Autodesk Inventor part; units mm, degrees
(part 2 of 2)
  measures "d114" diameter of A33
  measures "d115" diameter of A34
  measures "d116" diameter of A35
  measures "d117" diameter of A36
  measures "d118" diameter of A37
  measures "d119" diameter of A38
  measures "d120" diameter of A39
  measures "d121" diameter of A40
  measures "d122" diameter of A41
  measures "d123" diameter of A42
  measures "d124" diameter of A43
  measures "d125" diameter of A44
  measures "d126" diameter of A45
  measures "d127" diameter of A46
  measures "d128" diameter of A47
  measures "d129" diameter of A48
  measures "d130" diameter of A49
  measures "d131" diameter of A50
  measures "d132" diameter of A51
  measures "d133" diameter of A52
  measures "d134" diameter of A53
  measures "d135" diameter of A54
  measures "d136" diameter of A55
  measures "d137" diameter of A56
  measures "d138" diameter of A57
  measures "d139" diameter of A58
  measures "d140" diameter of A59
  measures "d141" diameter of A60
  measures "d142" diameter of A61
  measures "d143" diameter of A62
  measures "d144" diameter of A63
  measures "d145" diameter of A64
  measures "d146" diameter of A65
  measures "d147" diameter of A66
  measures "d148" diameter of A67
  measures "d149" diameter of A68
  measures "d150" diameter of A69
  measures "d151" diameter of A70
  measures "d152" diameter of A71
  measures "d155" diameter of A72
  measures "d156" diameter of A73
  measures "d264" diameter of A74
  measures "d265" diameter of A75
  measures "d267" distance between parallel lines of L17 L232
  measures "d268" diameter of A76
  measures "d269" diameter of A77
  measures "d270" diameter of A78
extrude "Extrusión2" add sketch "Boceto2" against normal up to surface (1.742 mm away)
sketch "Panel Shape" plane through (0, 0, 0) normal (0, 0, 1) x (1, 0, 0)
  line L0 (-22.8, -32.942) -> (-22.8, -37.5)
  arc A0 (-23.3, -38) -> (-22.8, -37.5) centre (-23.3, -37.5) ccw
  line L1 (-23.3, -38) -> (-29.8, -38)
  arc A1 (-30.3, -37.5) -> (-29.8, -38) centre (-29.8, -37.5) ccw
  line L2 (-30.3, -37.5) -> (-30.3, -31.2)
  arc A2 (-30.3, -31.2) -> (-30.8, -30.7) centre (-30.8, -31.2) ccw
  line L3 (-30.8, -30.7) -> (-76.8, -30.7)
  arc A3 (-76.8, -30.7) -> (-77.3, -31.2) centre (-76.8, -31.2) ccw
  line L4 (-77.3, -31.2) -> (-77.3, -49.2)
  arc A4 (-77.3, -49.2) -> (-75.3, -51.2) centre (-75.3, -49.2) ccw
  line L5 (-75.3, -51.2) -> (-71.048, -51.2)
  arc A5 (-65.048, -57.2) -> (-71.048, -51.2) centre (-71.048, -57.2) ccw
  line L6 (-65.048, -57.2) -> (-65.048, -62.7)
  arc A6 (-65.048, -62.7) -> (-63.048, -64.7) centre (-63.048, -62.7) ccw
  line L7 (-63.048, -64.7) -> (-30.8, -64.7)
  arc A7 (-30.8, -64.7) -> (-30.3, -64.2) centre (-30.8, -64.2) ccw
  line L8 (-30.3, -64.2) -> (-30.3, -59.8)
  arc A8 (-29.8, -59.3) -> (-30.3, -59.8) centre (-29.8, -59.8) ccw
  line L9 (-29.8, -59.3) -> (-23.3, -59.3)
  arc A9 (-22.8, -59.8) -> (-23.3, -59.3) centre (-23.3, -59.8) ccw
  line L10 (-22.8, -59.8) -> (-22.8, -62.458)
  arc A10 (-22.8, -62.458) -> (-22.3, -62.958) centre (-22.3, -62.458) ccw
  line L11 (-22.3, -62.958) -> (-16, -62.958)
  arc A11 (-16, -62.958) -> (-15.5, -62.458) centre (-16, -62.458) ccw
  line L12 (-15.5, -62.458) -> (-15.5, -60.4)
  arc A12 (25.5, -120.6) -> (26, -120.1) centre (25.5, -120.1) ccw
  line L13 (25.5, -120.6) -> (-25.5, -120.6)
  arc A13 (-26, -120.1) -> (-25.5, -120.6) centre (-25.5, -120.1) ccw
  line L14 (-26, -120.1) -> (-26, -66.6)
  arc A14 (-25.5, -66.1) -> (-26, -66.6) centre (-25.5, -66.6) ccw
  line L15 (-25.5, -66.1) -> (-16, -66.1)
  arc A15 (-15.5, -66.6) -> (-16, -66.1) centre (-16, -66.6) ccw
  line L16 (-15.5, -66.6) -> (-15.5, -72.9)
  arc A16 (-15.5, -72.9) -> (-15, -73.4) centre (-15, -72.9) ccw
  line L17 (-15, -59.9) -> (-13.5, -59.9)
  arc A17 (-13, -60.4) -> (-13.5, -59.9) centre (-13.5, -60.4) ccw
  line L18 (-13, -60.4) -> (-13, -72.9)
  arc A18 (-13.5, -73.4) -> (-13, -72.9) centre (-13.5, -72.9) ccw
  line L19 (-13.5, -73.4) -> (-15, -73.4)
  arc A19 (26, -73.9) -> (25.5, -73.4) centre (25.5, -73.9) ccw
  line L20 (26, -73.9) -> (26, -120.1)
  line L21 (7.4, 23.5) -> (7.4, 31.9)
  arc A20 (7.9, 32.4) -> (7.4, 31.9) centre (7.9, 31.9) ccw
  line L22 (7.9, 32.4) -> (12.55, 32.4)
  arc A21 (7.4, 23.5) -> (7.9, 23) centre (7.9, 23.5) ccw
  line L23 (7.9, 23) -> (25, 23)
  arc A22 (12.55, 32.4) -> (13.05, 32.9) centre (12.55, 32.9) ccw
  line L24 (13.05, 32.9) -> (13.05, 40.1)
  arc A23 (13.55, 40.6) -> (13.05, 40.1) centre (13.55, 40.1) ccw
  line L25 (13.55, 40.6) -> (36.8, 40.6)
  arc A24 (37.3, 40.1) -> (36.8, 40.6) centre (36.8, 40.1) ccw
  line L26 (37.3, 40.1) -> (37.3, 36)
  arc A25 (36.8, 35.5) -> (37.3, 36) centre (36.8, 36) ccw
  line L27 (36.8, 35.5) -> (34.4, 35.5)
  arc A26 (34.4, 35.5) -> (33.9, 35) centre (34.4, 35) ccw
  line L28 (33.9, 35) -> (33.9, 30.9)
  arc A27 (33.9, 30.9) -> (34.4, 30.4) centre (34.4, 30.9) ccw
  line L29 (38.9, 31.8) -> (38.9, 30.9)
  arc A28 (38.4, 30.4) -> (38.9, 30.9) centre (38.4, 30.9) ccw
  line L30 (38.4, 30.4) -> (34.4, 30.4)
  line L31 (77.3, 32.8) -> (77.3, 50.2)
  arc A29 (77.8, 50.7) -> (77.3, 50.2) centre (77.8, 50.2) ccw
  line L32 (77.8, 50.7) -> (79.8, 50.7)
  arc A30 (79.8, 50.7) -> (80.3, 51.2) centre (79.8, 51.2) ccw
  line L33 (80.3, 51.2) -> (80.3, 56.4)
  arc A31 (80.3, 56.4) -> (79.8, 56.9) centre (79.8, 56.4) ccw
  line L34 (79.8, 56.9) -> (58.9, 56.9)
  line L35 (54.4, 31.3) -> (57.9, 31.3)
  arc A32 (57.9, 31.3) -> (58.4, 31.8) centre (57.9, 31.8) ccw
  arc A33 (58.9, 32.3) -> (58.4, 31.8) centre (58.9, 31.8) ccw
  line L36 (58.9, 32.3) -> (76.8, 32.3)
  arc A34 (76.8, 32.3) -> (77.3, 32.8) centre (76.8, 32.8) ccw
  arc A35 (53.9, 31.8) -> (54.4, 31.3) centre (54.4, 31.8) ccw
  arc A36 (53.9, 31.8) -> (53.4, 32.3) centre (53.4, 31.8) ccw
  line L37 (53.4, 32.3) -> (39.4, 32.3)
  arc A37 (39.4, 32.3) -> (38.9, 31.8) centre (39.4, 31.8) ccw
  line L38 (36.8, 52) -> (13.55, 52)
  arc A38 (13.05, 52.5) -> (13.55, 52) centre (13.55, 52.5) ccw
  line L39 (13.05, 52.5) -> (13.05, 59.358)
  arc A39 (13.05, 59.358) -> (12.55, 59.858) centre (12.55, 59.358) ccw
  line L40 (12.55, 59.858) -> (-27.242, 59.858)
  arc A40 (36.8, 52) -> (37.3, 52.5) centre (36.8, 52.5) ccw
  line L41 (37.3, 52.5) -> (37.3, 53.2)
  arc A41 (-27.242, 59.858) -> (-27.742, 59.358) centre (-27.242, 59.358) ccw
  line L42 (-27.742, 59.358) -> (-27.742, 29.842)
  arc A42 (37.3, 53.2) -> (36.8, 53.7) centre (36.8, 53.2) ccw
  line L43 (36.8, 53.7) -> (34.4, 53.7)
  arc A43 (33.9, 54.2) -> (34.4, 53.7) centre (34.4, 54.2) ccw
  line L44 (33.9, 54.2) -> (33.9, 58.3)
  line L45 (-15, -26) -> (-13.5, -26)
  arc A44 (-13, -26.5) -> (-13.5, -26) centre (-13.5, -26.5) ccw
  line L46 (-13, -26.5) -> (-13, -35)
  arc A45 (-13.5, -35.5) -> (-13, -35) centre (-13.5, -35) ccw
  line L47 (-13.5, -35.5) -> (-15, -35.5)
  arc A46 (-15, -26) -> (-15.5, -26.5) centre (-15, -26.5) ccw
  line L48 (-15.5, -26.5) -> (-15.5, -28)
  arc A47 (-16, -28.5) -> (-15.5, -28) centre (-16, -28) ccw
  line L49 (-16, -28.5) -> (-25.5, -28.5)
  arc A48 (-26, -28) -> (-25.5, -28.5) centre (-25.5, -28) ccw
  line L50 (-26, -28) -> (-26, 25.5)
  arc A49 (-25.5, 26) -> (-26, 25.5) centre (-25.5, 25.5) ccw
  line L51 (-25.5, 26) -> (-20.6, 26)
  arc A50 (-20.1, 25.5) -> (-20.6, 26) centre (-20.6, 25.5) ccw
  line L52 (-20.1, 25.5) -> (-20.1, 23.5)
  arc A51 (-20.1, 23.5) -> (-19.6, 23) centre (-19.6, 23.5) ccw
  line L53 (-19.6, 32.4) -> (-18.3, 32.4)
  arc A52 (-17.8, 31.9) -> (-18.3, 32.4) centre (-18.3, 31.9) ccw
  line L54 (-17.8, 31.9) -> (-17.8, 23.5)
  arc A53 (-18.3, 23) -> (-17.8, 23.5) centre (-18.3, 23.5) ccw
  line L55 (-18.3, 23) -> (-19.6, 23)
  arc A54 (26, 22) -> (25, 23) centre (25, 22) ccw
  line L56 (26, 22) -> (26, -25.5)
  arc A55 (25.5, -26) -> (26, -25.5) centre (25.5, -25.5) ccw
  line L57 (-15.5, -35) -> (-15.5, -32.942)
  arc A56 (-15.5, -32.942) -> (-16, -32.442) centre (-16, -32.942) ccw
  line L58 (-16, -32.442) -> (-22.3, -32.442)
  arc A57 (-22.3, -32.442) -> (-22.8, -32.942) centre (-22.3, -32.942) ccw
  arc A58 (-15, -59.9) -> (-15.5, -60.4) centre (-15, -60.4) ccw
  arc A59 (25.5, -59.9) -> (26, -59.4) centre (25.5, -59.4) ccw
  line L59 (26, -59.4) -> (26, -36)
  arc A60 (26, -36) -> (25.5, -35.5) centre (25.5, -36) ccw
  arc A61 (-15.5, -35) -> (-15, -35.5) centre (-15, -35) ccw
  line L60 (25.5, -73.4) -> (25, -73.4)
  arc A62 (24.5, -72.9) -> (25, -73.4) centre (25, -72.9) ccw
  line L61 (24.5, -72.9) -> (24.5, -60.4)
  arc A63 (25, -59.9) -> (24.5, -60.4) centre (25, -60.4) ccw
  line L62 (25, -59.9) -> (25.5, -59.9)
  line L63 (24.5, -35) -> (24.5, -26.5)
  arc A64 (25, -26) -> (24.5, -26.5) centre (25, -26.5) ccw
  line L64 (25, -26) -> (25.5, -26)
  arc A65 (24.5, -35) -> (25, -35.5) centre (25, -35) ccw
  line L65 (25, -35.5) -> (25.5, -35.5)
  arc A66 (-27.742, 29.842) -> (-27.242, 29.342) centre (-27.242, 29.842) ccw
  line L66 (-27.242, 29.342) -> (-20.6, 29.342)
  arc A67 (-20.6, 29.342) -> (-20.1, 29.842) centre (-20.6, 29.842) ccw
  line L67 (-20.1, 29.842) -> (-20.1, 31.9)
  arc A68 (-19.6, 32.4) -> (-20.1, 31.9) centre (-19.6, 31.9) ccw
  arc A69 (34.4, 58.8) -> (33.9, 58.3) centre (34.4, 58.3) ccw
  arc A70 (58.4, 57.4) -> (58.9, 56.9) centre (58.9, 57.4) ccw
  arc A71 (58.4, 57.4) -> (57.9, 57.9) centre (57.9, 57.4) ccw
  line L68 (57.9, 57.9) -> (54.4, 57.9)
  arc A72 (54.4, 57.9) -> (53.9, 57.4) centre (54.4, 57.4) ccw
  arc A73 (53.4, 56.9) -> (53.9, 57.4) centre (53.4, 57.4) ccw
  line L69 (53.4, 56.9) -> (39.4, 56.9)
  arc A74 (38.9, 57.4) -> (39.4, 56.9) centre (39.4, 57.4) ccw
  line L70 (38.9, 57.4) -> (38.9, 58.3)
  arc A75 (38.9, 58.3) -> (38.4, 58.8) centre (38.4, 58.3) ccw
  line L71 (38.4, 58.8) -> (34.4, 58.8)
  circle A76 centre (-55.3, 51.4) radius 2.8
  circle A77 centre (58.3, 11.4) radius 2.8
  circle A78 centre (58.3, -43.6) radius 2.8
  circle A79 centre (58.3, -98.6) radius 2.8
  circle A80 centre (-55.3, -98.6) radius 2.8
  circle A81 centre (-55.3, -8.6) radius 2.8
  circle A82 centre (-20.3, -28.25) radius 0.25
  circle A83 centre (-19.3, -28.25) radius 0.25
  circle A84 centre (-18.3, -28.25) radius 0.25
  circle A85 centre (-19.3, -32.692) radius 0.25
  circle A86 centre (-18.3, -32.692) radius 0.25
  circle A87 centre (-20.3, -32.692) radius 0.25
  circle A88 centre (-28.25, -24.5) radius 0.25
  circle A89 centre (-25.75, -24.5) radius 0.25
  circle A90 centre (-25.75, -23.5) radius 0.25
  circle A91 centre (-25.75, -25.5) radius 0.25
  circle A92 centre (-28.25, -23.5) radius 0.25
  circle A93 centre (-28.25, -25.5) radius 0.25
  circle A94 centre (-28.25, -72.1) radius 0.25
  circle A95 centre (-25.75, -72.1) radius 0.25
  circle A96 centre (-25.75, -71.1) radius 0.25
  circle A97 centre (-25.75, -73.1) radius 0.25
  circle A98 centre (-28.25, -71.1) radius 0.25
  circle A99 centre (-28.25, -73.1) radius 0.25
  circle A100 centre (-36.3, -30.95) radius 0.25
  circle A101 centre (-36.3, -28.45) radius 0.25
  circle A102 centre (-37.3, -28.45) radius 0.25
  circle A103 centre (-35.3, -28.45) radius 0.25
  circle A104 centre (-37.3, -30.95) radius 0.25
  circle A105 centre (-35.3, -30.95) radius 0.25
  circle A106 centre (-71.3, -30.95) radius 0.25
  circle A107 centre (-71.3, -28.45) radius 0.25
  circle A108 centre (-72.3, -28.45) radius 0.25
  circle A109 centre (-70.3, -28.45) radius 0.25
  circle A110 centre (-72.3, -30.95) radius 0.25
  circle A111 centre (-70.3, -30.95) radius 0.25
  circle A112 centre (-59.05, -66.95) radius 0.25
  circle A113 centre (-59.05, -64.45) radius 0.25
  circle A114 centre (-60.05, -64.45) radius 0.25
  circle A115 centre (-58.05, -64.45) radius 0.25
  circle A116 centre (-60.05, -66.95) radius 0.25
  circle A117 centre (-58.05, -66.95) radius 0.25
  circle A118 centre (-36.3, -66.95) radius 0.25
  circle A119 centre (-36.3, -64.45) radius 0.25
  circle A120 centre (-37.3, -64.45) radius 0.25
  circle A121 centre (-35.3, -64.45) radius 0.25
  circle A122 centre (-37.3, -66.95) radius 0.25
  circle A123 centre (-35.3, -66.95) radius 0.25
  circle A124 centre (-19.3, -66.35) radius 0.25
  circle A125 centre (-19.3, -62.7) radius 0.25
  circle A126 centre (-20.3, -62.7) radius 0.25
  circle A127 centre (-18.3, -62.7) radius 0.25
  circle A128 centre (-20.3, -66.35) radius 0.25
  circle A129 centre (-18.3, -66.35) radius 0.25
  circle A130 centre (-25.75, -114.6) radius 0.25
  circle A131 centre (-28.25, -114.6) radius 0.25
  circle A132 centre (-28.25, -115.6) radius 0.25
  circle A133 centre (-28.25, -113.6) radius 0.25
  circle A134 centre (-25.75, -115.6) radius 0.25
  circle A135 centre (-25.75, -113.6) radius 0.25
  circle A136 centre (0, -120.35) radius 0.25
  circle A137 centre (0, -122.85) radius 0.25
  circle A138 centre (1, -122.85) radius 0.25
  circle A139 centre (-1, -122.85) radius 0.25
  circle A140 centre (1, -120.35) radius 0.25
  circle A141 centre (-1, -120.35) radius 0.25
  circle A142 centre (28.25, -114.6) radius 0.25
  circle A143 centre (25.75, -114.6) radius 0.25
  circle A144 centre (25.75, -115.6) radius 0.25
  circle A145 centre (25.75, -113.6) radius 0.25
  circle A146 centre (28.25, -115.6) radius 0.25
  circle A147 centre (28.25, -113.6) radius 0.25
  circle A148 centre (28.25, -82.8) radius 0.25
  circle A149 centre (25.75, -82.8) radius 0.25
  circle A150 centre (25.75, -83.8) radius 0.25
  circle A151 centre (25.75, -81.8) radius 0.25
  circle A152 centre (28.25, -83.8) radius 0.25
  circle A153 centre (28.25, -81.8) radius 0.25
  circle A154 centre (28.25, -20) radius 0.25
  circle A155 centre (25.75, -20) radius 0.25
  circle A156 centre (25.75, -21) radius 0.25
  circle A157 centre (25.75, -19) radius 0.25
  circle A158 centre (28.25, -21) radius 0.25
  circle A159 centre (28.25, -19) radius 0.25
  circle A160 centre (21, 22.75) radius 0.25
  circle A161 centre (21, 25.25) radius 0.25
  circle A162 centre (20, 25.25) radius 0.25
  circle A163 centre (22, 25.25) radius 0.25
  circle A164 centre (20, 22.75) radius 0.25
  circle A165 centre (22, 22.75) radius 0.25
  circle A166 centre (-25.75, 8.6) radius 0.25
  circle A167 centre (-28.25, 8.6) radius 0.25
  circle A168 centre (-28.25, 7.6) radius 0.25
  circle A169 centre (-28.25, 9.6) radius 0.25
  circle A170 centre (-25.75, 7.6) radius 0.25
  circle A171 centre (-25.75, 9.6) radius 0.25
  circle A172 centre (-27.492, 33.342) radius 0.25
  circle A173 centre (-27.492, 32.342) radius 0.25
  circle A174 centre (-27.492, 31.342) radius 0.25
  circle A175 centre (-29.992, 31.342) radius 0.25
  circle A176 centre (-29.992, 32.342) radius 0.25
  circle A177 centre (-29.992, 33.342) radius 0.25
  circle A178 centre (-29.992, 47.858) radius 0.25
  circle A179 centre (-27.492, 47.858) radius 0.25
  circle A180 centre (-29.992, 46.858) radius 0.25
  circle A181 centre (-29.992, 45.858) radius 0.25
  circle A182 centre (-27.492, 46.858) radius 0.25
  circle A183 centre (-27.492, 45.858) radius 0.25
  circle A184 centre (15.3, 36.6) radius 0.25
  circle A185 centre (15.3, 35.6) radius 0.25
  circle A186 centre (12.8, 34.6) radius 0.25
  circle A187 centre (12.8, 35.6) radius 0.25
  circle A188 centre (12.8, 36.6) radius 0.25
  circle A189 centre (15.3, 58) radius 0.25
  circle A190 centre (15.3, 57) radius 0.25
  circle A191 centre (15.3, 56) radius 0.25
  circle A192 centre (12.8, 56) radius 0.25
  circle A193 centre (12.8, 57) radius 0.25
  circle A194 centre (12.8, 58) radius 0.25
  circle A195 centre (28.25, -47.7) radius 0.25
  circle A196 centre (25.75, -47.7) radius 0.25
  circle A197 centre (25.75, -48.7) radius 0.25
  circle A198 centre (25.75, -46.7) radius 0.25
  circle A199 centre (28.25, -48.7) radius 0.25
  circle A200 centre (28.25, -46.7) radius 0.25
  circle A201 centre (25.75, -49.7) radius 0.25
  circle A202 centre (25.75, -45.7) radius 0.25
  circle A203 centre (28.25, -45.7) radius 0.25
  circle A204 centre (28.25, -49.7) radius 0.25
  circle A205 centre (47.7, 61.05) radius 0.25
  circle A206 centre (47.7, 56.65) radius 0.25
  circle A207 centre (48.7, 56.65) radius 0.25
  circle A208 centre (46.7, 56.65) radius 0.25
  circle A209 centre (48.7, 61.05) radius 0.25
  circle A210 centre (46.7, 61.05) radius 0.25
  circle A211 centre (69.7, 61.05) radius 0.25
  circle A212 centre (69.7, 56.65) radius 0.25
  circle A213 centre (70.7, 56.65) radius 0.25
  circle A214 centre (68.7, 56.65) radius 0.25
  circle A215 centre (70.7, 61.05) radius 0.25
  circle A216 centre (68.7, 61.05) radius 0.25
  circle A217 centre (69.7, 32.55) radius 0.25
  circle A218 centre (69.7, 28.15) radius 0.25
  circle A219 centre (70.7, 28.15) radius 0.25
  circle A220 centre (68.7, 28.15) radius 0.25
  circle A221 centre (70.7, 32.55) radius 0.25
  circle A222 centre (68.7, 32.55) radius 0.25
  circle A223 centre (47.7, 32.55) radius 0.25
  circle A224 centre (47.7, 28.15) radius 0.25
  circle A225 centre (48.7, 28.15) radius 0.25
  circle A226 centre (46.7, 28.15) radius 0.25
  circle A227 centre (48.7, 32.55) radius 0.25
  circle A228 centre (46.7, 32.55) radius 0.25
  circle A229 centre (-5.6, 62.108) radius 0.25
  circle A230 centre (-5.6, 59.608) radius 0.25
  circle A231 centre (-4.6, 59.608) radius 0.25
  circle A232 centre (-6.6, 59.608) radius 0.25
  circle A233 centre (-4.6, 62.108) radius 0.25
  circle A234 centre (-6.6, 62.108) radius 0.25
  circle A235 centre (23.035, -105.13) radius 0.37
  circle A236 centre (23.035, -106.4) radius 0.37
  circle A237 centre (23.035, -107.67) radius 0.37
  circle A238 centre (21.765, -105.13) radius 0.37
  circle A239 centre (21.765, -106.4) radius 0.37
  circle A240 centre (21.765, -107.67) radius 0.37
  circle A241 centre (23.035, -103.86) radius 0.37
  circle A242 centre (21.765, -103.86) radius 0.37
  circle A243 centre (23.035, -108.94) radius 0.37
  circle A244 centre (21.765, -108.94) radius 0.37
  circle A245 centre (-11.095, -17.035) radius 0.37
  circle A246 centre (-12.365, -17.035) radius 0.37
  circle A247 centre (-11.095, -15.765) radius 0.37
  circle A248 centre (-12.365, -15.765) radius 0.37
  circle A249 centre (-9.825, -17.035) radius 0.37
  circle A250 centre (-9.825, -15.765) radius 0.37
  circle A251 centre (-14.905, -17.035) radius 0.37
  circle A252 centre (-16.175, -17.035) radius 0.37
  circle A253 centre (-14.905, -15.765) radius 0.37
  circle A254 centre (-16.175, -15.765) radius 0.37
  circle A255 centre (-13.635, -17.035) radius 0.37
  circle A256 centre (-13.635, -15.765) radius 0.37
  circle A257 centre (21.465, -50.97) radius 0.37
  circle A258 centre (21.465, -49.7) radius 0.37
  circle A259 centre (21.465, -48.43) radius 0.37
  circle A260 centre (22.735, -50.97) radius 0.37
  circle A261 centre (22.735, -49.7) radius 0.37
  circle A262 centre (22.735, -48.43) radius 0.37
  circle A263 centre (21.465, -52.24) radius 0.37
  circle A264 centre (22.735, -52.24) radius 0.37
  circle A265 centre (21.465, -47.16) radius 0.37
  circle A266 centre (22.735, -47.16) radius 0.37
  circle A267 centre (73, 53.6) radius 1.5
  circle A268 centre (44.6, 35.6) radius 1.5
  circle A269 centre (44.6, 53.6) radius 1.5
  circle A270 centre (73, 35.6) radius 1.5
  circle A271 centre (15.3, 34.6) radius 0.25
  circle A272 centre (-36.6, -61.378) radius 2
  circle A273 centre (-36.6, -34.022) radius 2
  circle A274 centre (-19.1, -36.062) radius 2
  circle A275 centre (-23.092, 32.962) radius 2
  circle A276 centre (-9.192, 56.238) radius 2
  circle A277 centre (36.4, 56.256) radius 2
  circle A278 centre (78.021, 53.178) radius 2
  circle A279 centre (36.4, 32.98) radius 2
  circle A280 centre (56.15, 55.6) radius 2
  circle A281 centre (56.15, 33.6) radius 2
  circle A282 centre (-19.1, -59.338) radius 2
  circle A283 centre (-67.2, -34.022) radius 2
  circle A284 centre (-82.3, 64.858) radius 1.65
  circle A285 centre (85.3, 64.858) radius 1.65
  circle A286 centre (85.3, -125.6) radius 1.65
  circle A287 centre (-82.3, -125.6) radius 1.65
  arc A288 (31.4, 53.4) -> (31.9, 53.9) centre (31.4, 53.9) ccw
  line L72 (38.4, 58.8) -> (34.4, 58.8)
  line L73 (-76.8, -30.7) -> (-73.3, -30.7)
  line L74 (-79.3, -52.2) -> (-79.3, -29.7)
  arc A289 (-78.3, -28.7) -> (-79.3, -29.7) centre (-78.3, -29.7) ccw
  line L75 (-78.3, -28.7) -> (-73.3, -28.7)
  arc A290 (-73.3, -30.7) -> (-73.3, -28.7) centre (-73.3, -29.7) ccw
  arc A291 (-69.3, -28.7) -> (-69.3, -30.7) centre (-69.3, -29.7) ccw
  line L76 (-69.3, -28.7) -> (-38.3, -28.7)
  arc A292 (-38.3, -30.7) -> (-38.3, -28.7) centre (-38.3, -29.7) ccw
  arc A293 (-34.3, -28.7) -> (-34.3, -30.7) centre (-34.3, -29.7) ccw
  line L77 (-34.3, -28.7) -> (-28.5, -28.7)
  arc A294 (-28.5, -28.7) -> (-28, -28.2) centre (-28.5, -28.2) ccw
  line L78 (-28, -28.2) -> (-28, -26.3)
  arc A295 (-26, -26.3) -> (-28, -26.3) centre (-27, -26.3) ccw
  arc A296 (-28, -22.5) -> (-26, -22.5) centre (-27, -22.5) ccw
  line L79 (-28, -22.5) -> (-28, 6.6)
  arc A297 (-26, 6.6) -> (-28, 6.6) centre (-27, 6.6) ccw
  arc A298 (-28, 10.6) -> (-26, 10.6) centre (-27, 10.6) ccw
  line L80 (-28, 10.6) -> (-28, 26.842)
  arc A299 (-28, 26.842) -> (-28.5, 27.342) centre (-28.5, 26.842) ccw
  line L81 (-28.5, 27.342) -> (-28.742, 27.342)
  arc A300 (-29.742, 28.342) -> (-28.742, 27.342) centre (-28.742, 28.342) ccw
  line L82 (-29.742, 28.342) -> (-29.742, 30.342)
  arc A301 (-27.742, 30.342) -> (-29.742, 30.342) centre (-28.742, 30.342) ccw
  arc A302 (-29.742, 34.342) -> (-27.742, 34.342) centre (-28.742, 34.342) ccw
  line L83 (-29.742, 34.342) -> (-29.742, 44.858)
  arc A303 (-27.742, 44.858) -> (-29.742, 44.858) centre (-28.742, 44.858) ccw
  arc A304 (-29.742, 48.858) -> (-27.742, 48.858) centre (-28.742, 48.858) ccw
  line L84 (-29.742, 48.858) -> (-29.742, 60.858)
  arc A305 (-28.742, 61.858) -> (-29.742, 60.858) centre (-28.742, 60.858) ccw
  arc A306 (15.05, 60.858) -> (14.05, 61.858) centre (14.05, 60.858) ccw
  line L85 (15.05, 60.858) -> (15.05, 59)
  arc A307 (13.05, 59) -> (15.05, 59) centre (14.05, 59) ccw
  line L86 (31.4, 53.4) -> (15.55, 53.4)
  arc A308 (15.05, 53.9) -> (15.55, 53.4) centre (15.55, 53.9) ccw
  line L87 (15.05, 53.9) -> (15.05, 55)
  arc A309 (15.05, 55) -> (14.05, 56) centre (14.05, 55) ccw
  arc A310 (14.05, 56) -> (13.05, 55) centre (14.05, 55) ccw
  line L88 (13.05, 55) -> (13.05, 52.5)
  arc A311 (31.9, 29.4) -> (32.9, 28.4) centre (32.9, 29.4) ccw
  line L89 (31.9, 53.9) -> (31.9, 59.8)
  arc A312 (32.9, 60.8) -> (31.9, 59.8) centre (32.9, 59.8) ccw
  line L90 (32.9, 60.8) -> (45.7, 60.8)
  arc A313 (46.7, 59.8) -> (45.7, 60.8) centre (45.7, 59.8) ccw
  line L91 (46.7, 59.8) -> (46.7, 57.9)
  arc A314 (45.7, 56.9) -> (46.7, 57.9) centre (45.7, 57.9) ccw
  arc A315 (48.7, 57.9) -> (49.7, 56.9) centre (49.7, 57.9) ccw
  line L92 (48.7, 57.9) -> (48.7, 59.8)
  arc A316 (49.7, 60.8) -> (48.7, 59.8) centre (49.7, 59.8) ccw
  line L93 (49.7, 60.8) -> (67.7, 60.8)
  arc A317 (68.7, 59.8) -> (67.7, 60.8) centre (67.7, 59.8) ccw
  line L94 (68.7, 59.8) -> (68.7, 57.9)
  arc A318 (67.7, 56.9) -> (68.7, 57.9) centre (67.7, 57.9) ccw
  arc A319 (70.7, 57.9) -> (71.7, 56.9) centre (71.7, 57.9) ccw
  line L95 (70.7, 57.9) -> (70.7, 59.8)
  arc A320 (71.7, 60.8) -> (70.7, 59.8) centre (71.7, 59.8) ccw
  line L96 (71.7, 60.8) -> (81.3, 60.8)
  arc A321 (82.3, 59.8) -> (81.3, 60.8) centre (81.3, 59.8) ccw
  line L97 (82.3, 59.8) -> (82.3, 49.7)
  arc A322 (81.3, 48.7) -> (82.3, 49.7) centre (81.3, 49.7) ccw
  line L98 (81.3, 48.7) -> (80.3, 48.7)
  arc A323 (80.3, 48.7) -> (79.3, 47.7) centre (80.3, 47.7) ccw
  line L99 (79.3, 47.7) -> (79.3, 29.4)
  arc A324 (78.3, 28.4) -> (79.3, 29.4) centre (78.3, 29.4) ccw
  line L100 (78.3, 28.4) -> (71.7, 28.4)
  arc A325 (70.7, 29.4) -> (71.7, 28.4) centre (71.7, 29.4) ccw
  line L101 (70.7, 29.4) -> (70.7, 31.3)
  arc A326 (71.7, 32.3) -> (70.7, 31.3) centre (71.7, 31.3) ccw
  arc A327 (68.7, 31.3) -> (67.7, 32.3) centre (67.7, 31.3) ccw
  line L102 (68.7, 31.3) -> (68.7, 29.4)
  arc A328 (67.7, 28.4) -> (68.7, 29.4) centre (67.7, 29.4) ccw
  line L103 (67.7, 28.4) -> (49.7, 28.4)
  arc A329 (48.7, 29.4) -> (49.7, 28.4) centre (49.7, 29.4) ccw
  line L104 (48.7, 29.4) -> (48.7, 31.3)
  arc A330 (49.7, 32.3) -> (48.7, 31.3) centre (49.7, 31.3) ccw
  arc A331 (46.7, 31.3) -> (45.7, 32.3) centre (45.7, 31.3) ccw
  line L105 (46.7, 31.3) -> (46.7, 29.4)
  arc A332 (45.7, 28.4) -> (46.7, 29.4) centre (45.7, 29.4) ccw
  line L106 (45.7, 28.4) -> (32.9, 28.4)
  line L107 (-69.3, -30.7) -> (-38.3, -30.7)
  line L108 (31.9, 29.4) -> (31.9, 37.9)
  arc A333 (31.9, 37.9) -> (31.4, 38.4) centre (31.4, 37.9) ccw
  line L109 (31.4, 38.4) -> (15.55, 38.4)
  arc A334 (15.55, 38.4) -> (15.05, 37.9) centre (15.55, 37.9) ccw
  line L110 (15.05, 37.9) -> (15.05, 37.6)
  arc A335 (14.05, 36.6) -> (15.05, 37.6) centre (14.05, 37.6) ccw
  arc A336 (13.05, 37.6) -> (14.05, 36.6) centre (14.05, 37.6) ccw
  line L111 (13.05, 37.6) -> (13.05, 40.1)
  arc A337 (15.05, 33.6) -> (13.05, 33.6) centre (14.05, 33.6) ccw
  line L112 (15.05, 33.6) -> (15.058, 25.5)
  arc A338 (15.058, 25.5) -> (15.558, 25) centre (15.558, 25.5) ccw
  line L113 (15.558, 25) -> (19, 25)
  arc A339 (19, 23) -> (19, 25) centre (19, 24) ccw
  arc A340 (23, 25) -> (23, 23) centre (23, 24) ccw
  line L114 (23, 25) -> (27, 25)
  arc A341 (28, 24) -> (27, 25) centre (27, 24) ccw
  line L115 (28, 24) -> (28, -18)
  arc A342 (26, -18) -> (28, -18) centre (27, -18) ccw
  arc A343 (28, -22) -> (26, -22) centre (27, -22) ccw
  line L116 (28, -22) -> (28, -44.7)
  arc A344 (26, -44.7) -> (28, -44.7) centre (27, -44.7) ccw
  arc A345 (28, -50.7) -> (26, -50.7) centre (27, -50.7) ccw
  line L117 (28, -50.7) -> (28, -80.8)
  arc A346 (26, -80.8) -> (28, -80.8) centre (27, -80.8) ccw
  arc A347 (28, -84.8) -> (26, -84.8) centre (27, -84.8) ccw
  line L118 (28, -84.8) -> (28, -112.6)
  arc A348 (26, -112.6) -> (28, -112.6) centre (27, -112.6) ccw
  arc A349 (28, -116.6) -> (26, -116.6) centre (27, -116.6) ccw
  line L119 (28, -116.6) -> (28, -121.6)
  arc A350 (27, -122.6) -> (28, -121.6) centre (27, -121.6) ccw
  line L120 (27, -122.6) -> (2, -122.6)
  arc A351 (2, -120.6) -> (2, -122.6) centre (2, -121.6) ccw
  arc A352 (-2, -122.6) -> (-2, -120.6) centre (-2, -121.6) ccw
  line L121 (-2, -122.6) -> (-27, -122.6)
  arc A353 (-28, -121.6) -> (-27, -122.6) centre (-27, -121.6) ccw
  line L122 (-28, -121.6) -> (-28, -116.6)
  arc A354 (-26, -116.6) -> (-28, -116.6) centre (-27, -116.6) ccw
  arc A355 (-28, -112.6) -> (-26, -112.6) centre (-27, -112.6) ccw
  line L123 (-28, -112.6) -> (-28, -74.1)
  arc A356 (-26, -74.1) -> (-28, -74.1) centre (-27, -74.1) ccw
  arc A357 (-28, -70.1) -> (-26, -70.1) centre (-27, -70.1) ccw
  line L124 (-28, -70.1) -> (-28, -67.2)
  arc A358 (-28, -67.2) -> (-28.5, -66.7) centre (-28.5, -67.2) ccw
  line L125 (-28.5, -66.7) -> (-34.3, -66.7)
  arc A359 (-34.3, -64.7) -> (-34.3, -66.7) centre (-34.3, -65.7) ccw
  arc A360 (-38.3, -66.7) -> (-38.3, -64.7) centre (-38.3, -65.7) ccw
  line L126 (-38.3, -66.7) -> (-57.048, -66.7)
  arc A361 (-57.048, -64.7) -> (-57.048, -66.7) centre (-57.048, -65.7) ccw
  arc A362 (-61.048, -66.7) -> (-61.048, -64.7) centre (-61.048, -65.7) ccw
  line L127 (-61.048, -66.7) -> (-66.048, -66.7)
  arc A363 (-67.048, -65.7) -> (-66.048, -66.7) centre (-66.048, -65.7) ccw
  line L128 (-67.048, -65.7) -> (-67.048, -57.2)
  arc A364 (-67.048, -57.2) -> (-71.048, -53.2) centre (-71.048, -57.2) ccw
  line L129 (-71.048, -53.2) -> (-78.3, -53.2)
  arc A365 (-79.3, -52.2) -> (-78.3, -53.2) centre (-78.3, -52.2) ccw
  line L130 (-20.3, -29.5) -> (-20.3, -31.442)
  arc A366 (-21.3, -32.442) -> (-20.3, -31.442) centre (-21.3, -31.442) ccw
  arc A367 (-18.3, -31.442) -> (-17.3, -32.442) centre (-17.3, -31.442) ccw
  line L131 (-18.3, -31.442) -> (-18.3, -29.5)
  arc A368 (-17.3, -28.5) -> (-18.3, -29.5) centre (-17.3, -29.5) ccw
  arc A369 (-20.3, -29.5) -> (-21.3, -28.5) centre (-21.3, -29.5) ccw
  line L132 (-20.3, -63.958) -> (-20.3, -65.1)
  arc A370 (-21.3, -66.1) -> (-20.3, -65.1) centre (-21.3, -65.1) ccw
  arc A371 (-18.3, -65.1) -> (-17.3, -66.1) centre (-17.3, -65.1) ccw
  line L133 (-18.3, -65.1) -> (-18.3, -63.958)
  arc A372 (-17.3, -62.958) -> (-18.3, -63.958) centre (-17.3, -63.958) ccw
  arc A373 (-20.3, -63.958) -> (-21.3, -62.958) centre (-21.3, -63.958) ccw
  line L134 (-22.8, -32.942) -> (-22.8, -37.5)
  arc A374 (-23.3, -38) -> (-22.8, -37.5) centre (-23.3, -37.5) ccw
  line L135 (-23.3, -38) -> (-29.8, -38)
  arc A375 (-30.3, -37.5) -> (-29.8, -38) centre (-29.8, -37.5) ccw
  line L136 (-30.3, -37.5) -> (-30.3, -31.2)
  arc A376 (-30.3, -31.2) -> (-30.8, -30.7) centre (-30.8, -31.2) ccw
  arc A377 (-76.8, -30.7) -> (-77.3, -31.2) centre (-76.8, -31.2) ccw
  line L137 (-77.3, -31.2) -> (-77.3, -49.2)
  arc A378 (-77.3, -49.2) -> (-75.3, -51.2) centre (-75.3, -49.2) ccw
  line L138 (-75.3, -51.2) -> (-71.048, -51.2)
  arc A379 (-65.048, -57.2) -> (-71.048, -51.2) centre (-71.048, -57.2) ccw
  line L139 (-65.048, -57.2) -> (-65.048, -62.7)
  arc A380 (-65.048, -62.7) -> (-63.048, -64.7) centre (-63.048, -62.7) ccw
  arc A381 (-30.8, -64.7) -> (-30.3, -64.2) centre (-30.8, -64.2) ccw
  line L140 (-30.3, -64.2) -> (-30.3, -59.8)
  arc A382 (-29.8, -59.3) -> (-30.3, -59.8) centre (-29.8, -59.8) ccw
  line L141 (-29.8, -59.3) -> (-23.3, -59.3)
  arc A383 (-22.8, -59.8) -> (-23.3, -59.3) centre (-23.3, -59.8) ccw
  line L142 (-22.8, -59.8) -> (-22.8, -62.458)
  arc A384 (-22.8, -62.458) -> (-22.3, -62.958) centre (-22.3, -62.458) ccw
  arc A385 (-16, -62.958) -> (-15.5, -62.458) centre (-16, -62.458) ccw
  line L143 (-15.5, -62.458) -> (-15.5, -60.4)
  arc A386 (25.5, -120.6) -> (26, -120.1) centre (25.5, -120.1) ccw
  arc A387 (-26, -120.1) -> (-25.5, -120.6) centre (-25.5, -120.1) ccw
  arc A388 (-25.5, -66.1) -> (-26, -66.6) centre (-25.5, -66.6) ccw
  arc A389 (-15.5, -66.6) -> (-16, -66.1) centre (-16, -66.6) ccw
  line L144 (-15.5, -66.6) -> (-15.5, -72.9)
  arc A390 (-15.5, -72.9) -> (-15, -73.4) centre (-15, -72.9) ccw
  line L145 (-15, -59.9) -> (-13.5, -59.9)
  arc A391 (-13, -60.4) -> (-13.5, -59.9) centre (-13.5, -60.4) ccw
  line L146 (-13, -60.4) -> (-13, -72.9)
  arc A392 (-13.5, -73.4) -> (-13, -72.9) centre (-13.5, -72.9) ccw
  line L147 (-13.5, -73.4) -> (-15, -73.4)
  arc A393 (26, -73.9) -> (25.5, -73.4) centre (25.5, -73.9) ccw
  line L148 (7.4, 23.5) -> (7.4, 31.9)
  arc A394 (7.9, 32.4) -> (7.4, 31.9) centre (7.9, 31.9) ccw
  line L149 (7.9, 32.4) -> (12.55, 32.4)
  arc A395 (7.4, 23.5) -> (7.9, 23) centre (7.9, 23.5) ccw
  arc A396 (12.55, 32.4) -> (13.05, 32.9) centre (12.55, 32.9) ccw
  arc A397 (13.55, 40.6) -> (13.05, 40.1) centre (13.55, 40.1) ccw
  line L150 (13.55, 40.6) -> (36.8, 40.6)
  arc A398 (37.3, 40.1) -> (36.8, 40.6) centre (36.8, 40.1) ccw
  line L151 (37.3, 40.1) -> (37.3, 36)
  arc A399 (36.8, 35.5) -> (37.3, 36) centre (36.8, 36) ccw
  line L152 (36.8, 35.5) -> (34.4, 35.5)
  arc A400 (34.4, 35.5) -> (33.9, 35) centre (34.4, 35) ccw
  line L153 (33.9, 35) -> (33.9, 30.9)
  line L154 (-61.048, -64.7) -> (-63.048, -64.7)
  line L155 (-38.3, -64.7) -> (-57.048, -64.7)
  line L156 (-34.3, -64.7) -> (-30.8, -64.7)
  line L157 (-25.5, -66.1) -> (-21.3, -66.1)
  line L158 (-17.3, -66.1) -> (-16, -66.1)
  line L159 (-22.3, -62.958) -> (-21.3, -62.958)
  line L160 (-17.3, -62.958) -> (-16, -62.958)
  line L161 (-26, -112.6) -> (-26, -74.1)
  line L162 (-26, -120.1) -> (-26, -116.6)
  line L163 (-2, -120.6) -> (-25.5, -120.6)
  line L164 (25.5, -120.6) -> (2, -120.6)
  line L165 (26, -116.6) -> (26, -120.1)
  line L166 (26, -84.8) -> (26, -112.6)
  line L167 (26, -73.9) -> (26, -80.8)
  line L168 (26, -50.7) -> (26, -59.4)
  line L169 (-26, -70.1) -> (-26, -66.6)
  line L170 (-34.3, -30.7) -> (-30.8, -30.7)
  line L171 (-26, -28) -> (-26, -26.3)
  line L172 (-25.5, -28.5) -> (-21.3, -28.5)
  line L173 (-22.3, -32.442) -> (-21.3, -32.442)
  line L174 (-17.3, -32.442) -> (-16, -32.442)
  line L175 (-17.3, -28.5) -> (-16, -28.5)
  line L176 (26, -36) -> (26, -44.7)
  line L177 (26, -22) -> (26, -25.5)
  line L178 (26, 22) -> (26, -18)
  line L179 (23, 23) -> (25, 23)
  line L180 (7.9, 23) -> (19, 23)
  line L181 (13.05, 32.9) -> (13.05, 33.6)
  line L182 (-26, -22.5) -> (-26, 6.6)
  line L183 (-26, 10.6) -> (-26, 25.5)
  line L184 (-27.742, 29.842) -> (-27.742, 30.342)
  line L185 (-27.742, 34.342) -> (-27.742, 44.858)
  line L186 (-27.742, 48.858) -> (-27.742, 59.358)
  line L187 (13.05, 59.358) -> (13.05, 59)
  line L188 (39.4, 56.9) -> (45.7, 56.9)
  line L189 (49.7, 56.9) -> (53.4, 56.9)
  line L190 (58.9, 56.9) -> (67.7, 56.9)
  line L191 (71.7, 56.9) -> (79.8, 56.9)
  line L192 (45.7, 32.3) -> (39.4, 32.3)
  line L193 (53.4, 32.3) -> (49.7, 32.3)
  line L194 (67.7, 32.3) -> (58.9, 32.3)
  line L195 (76.8, 32.3) -> (71.7, 32.3)
  arc A401 (-3.6, 61.858) -> (-3.6, 59.858) centre (-3.6, 60.858) ccw
  arc A402 (-7.6, 59.858) -> (-7.6, 61.858) centre (-7.6, 60.858) ccw
  arc A403 (33.9, 30.9) -> (34.4, 30.4) centre (34.4, 30.9) ccw
  line L196 (14.05, 61.858) -> (-3.6, 61.858)
  line L197 (12.55, 59.858) -> (-3.6, 59.858)
  line L198 (-7.6, 61.858) -> (-28.742, 61.858)
  line L199 (-7.6, 59.858) -> (-27.242, 59.858)
  line L200 (38.9, 31.8) -> (38.9, 30.9)
  arc A404 (38.4, 30.4) -> (38.9, 30.9) centre (38.4, 30.9) ccw
  line L201 (38.4, 30.4) -> (34.4, 30.4)
  line L202 (77.3, 32.8) -> (77.3, 50.2)
  arc A405 (77.8, 50.7) -> (77.3, 50.2) centre (77.8, 50.2) ccw
  line L203 (77.8, 50.7) -> (79.8, 50.7)
  arc A406 (79.8, 50.7) -> (80.3, 51.2) centre (79.8, 51.2) ccw
  line L204 (80.3, 51.2) -> (80.3, 56.4)
  arc A407 (80.3, 56.4) -> (79.8, 56.9) centre (79.8, 56.4) ccw
  line L205 (54.4, 31.3) -> (57.9, 31.3)
  arc A408 (57.9, 31.3) -> (58.4, 31.8) centre (57.9, 31.8) ccw
  arc A409 (58.9, 32.3) -> (58.4, 31.8) centre (58.9, 31.8) ccw
  arc A410 (76.8, 32.3) -> (77.3, 32.8) centre (76.8, 32.8) ccw
  arc A411 (53.9, 31.8) -> (54.4, 31.3) centre (54.4, 31.8) ccw
  arc A412 (53.9, 31.8) -> (53.4, 32.3) centre (53.4, 31.8) ccw
  arc A413 (39.4, 32.3) -> (38.9, 31.8) centre (39.4, 31.8) ccw
  line L206 (36.8, 52) -> (13.55, 52)
  arc A414 (13.05, 52.5) -> (13.55, 52) centre (13.55, 52.5) ccw
  arc A415 (13.05, 59.358) -> (12.55, 59.858) centre (12.55, 59.358) ccw
  arc A416 (36.8, 52) -> (37.3, 52.5) centre (36.8, 52.5) ccw
  line L207 (37.3, 52.5) -> (37.3, 53.2)
  arc A417 (-27.242, 59.858) -> (-27.742, 59.358) centre (-27.242, 59.358) ccw
  arc A418 (37.3, 53.2) -> (36.8, 53.7) centre (36.8, 53.2) ccw
  line L208 (36.8, 53.7) -> (34.4, 53.7)
  arc A419 (33.9, 54.2) -> (34.4, 53.7) centre (34.4, 54.2) ccw
  line L209 (33.9, 54.2) -> (33.9, 58.3)
  line L210 (-15, -26) -> (-13.5, -26)
  arc A420 (-13, -26.5) -> (-13.5, -26) centre (-13.5, -26.5) ccw
  line L211 (-13, -26.5) -> (-13, -35)
  arc A421 (-13.5, -35.5) -> (-13, -35) centre (-13.5, -35) ccw
  line L212 (-13.5, -35.5) -> (-15, -35.5)
  arc A422 (-15, -26) -> (-15.5, -26.5) centre (-15, -26.5) ccw
  line L213 (-15.5, -26.5) -> (-15.5, -28)
  arc A423 (-16, -28.5) -> (-15.5, -28) centre (-16, -28) ccw
  arc A424 (-26, -28) -> (-25.5, -28.5) centre (-25.5, -28) ccw
  arc A425 (-25.5, 26) -> (-26, 25.5) centre (-25.5, 25.5) ccw
  line L214 (-25.5, 26) -> (-20.6, 26)
  arc A426 (-20.1, 25.5) -> (-20.6, 26) centre (-20.6, 25.5) ccw
  line L215 (-20.1, 25.5) -> (-20.1, 23.5)
  arc A427 (-20.1, 23.5) -> (-19.6, 23) centre (-19.6, 23.5) ccw
  line L216 (-19.6, 32.4) -> (-18.3, 32.4)
  arc A428 (-17.8, 31.9) -> (-18.3, 32.4) centre (-18.3, 31.9) ccw
  line L217 (-17.8, 31.9) -> (-17.8, 23.5)
  arc A429 (-18.3, 23) -> (-17.8, 23.5) centre (-18.3, 23.5) ccw
  line L218 (-18.3, 23) -> (-19.6, 23)
  arc A430 (26, 22) -> (25, 23) centre (25, 22) ccw
  arc A431 (25.5, -26) -> (26, -25.5) centre (25.5, -25.5) ccw
  line L219 (-15.5, -35) -> (-15.5, -32.942)
  arc A432 (-15.5, -32.942) -> (-16, -32.442) centre (-16, -32.942) ccw
  arc A433 (-22.3, -32.442) -> (-22.8, -32.942) centre (-22.3, -32.942) ccw
  arc A434 (-15, -59.9) -> (-15.5, -60.4) centre (-15, -60.4) ccw
  arc A435 (25.5, -59.9) -> (26, -59.4) centre (25.5, -59.4) ccw
  arc A436 (26, -36) -> (25.5, -35.5) centre (25.5, -36) ccw
  arc A437 (-15.5, -35) -> (-15, -35.5) centre (-15, -35) ccw
  line L220 (25.5, -73.4) -> (25, -73.4)
  arc A438 (24.5, -72.9) -> (25, -73.4) centre (25, -72.9) ccw
  line L221 (24.5, -72.9) -> (24.5, -60.4)
  arc A439 (25, -59.9) -> (24.5, -60.4) centre (25, -60.4) ccw
  line L222 (25, -59.9) -> (25.5, -59.9)
  line L223 (24.5, -35) -> (24.5, -26.5)
  arc A440 (25, -26) -> (24.5, -26.5) centre (25, -26.5) ccw
  line L224 (25, -26) -> (25.5, -26)
  arc A441 (24.5, -35) -> (25, -35.5) centre (25, -35) ccw
  line L225 (25, -35.5) -> (25.5, -35.5)
  arc A442 (-27.742, 29.842) -> (-27.242, 29.342) centre (-27.242, 29.842) ccw
  line L226 (-27.242, 29.342) -> (-20.6, 29.342)
  arc A443 (-20.6, 29.342) -> (-20.1, 29.842) centre (-20.6, 29.842) ccw
  line L227 (-20.1, 29.842) -> (-20.1, 31.9)
  arc A444 (-19.6, 32.4) -> (-20.1, 31.9) centre (-19.6, 31.9) ccw
  arc A445 (34.4, 58.8) -> (33.9, 58.3) centre (34.4, 58.3) ccw
  arc A446 (58.4, 57.4) -> (58.9, 56.9) centre (58.9, 57.4) ccw
  arc A447 (58.4, 57.4) -> (57.9, 57.9) centre (57.9, 57.4) ccw
  line L228 (57.9, 57.9) -> (54.4, 57.9)
  arc A448 (54.4, 57.9) -> (53.9, 57.4) centre (54.4, 57.4) ccw
  arc A449 (53.4, 56.9) -> (53.9, 57.4) centre (53.4, 57.4) ccw
  arc A450 (38.9, 57.4) -> (39.4, 56.9) centre (39.4, 57.4) ccw
  line L229 (38.9, 57.4) -> (38.9, 58.3)
  arc A451 (38.9, 58.3) -> (38.4, 58.8) centre (38.4, 58.3) ccw
  line L230 (-87.3, -130.6) -> (-87.3, 69.858)
  line L231 (90.3, 69.858) -> (90.3, -130.6)
  line L232 (90.3, -130.6) -> (-87.3, -130.6)
  line L233 (-87.3, 69.858) -> (90.3, 69.858)
  point P0 (0, 0)
  point P1 (90.3, 69.858)
  constraints: 480 point on circle, 468 end point, 452 centre point
sketch "Boceto3" plane through (0, 0, 0) normal (0, 0, 1) x (1, 0, 0)
  line L0 (-87.3, 69.858) -> (90.3, 69.858) construction
  line L1 (-87.3, -130.6) -> (-87.3, 69.858) construction
  line L2 (90.3, 69.858) -> (90.3, -130.6) construction
  line L3 (90.3, -130.6) -> (-87.3, -130.6) construction
  point P0 (0, 0)
  point P1 (-82.3, 64.858)
  point P2 (85.3, 64.858)
  point P3 (85.3, -125.6)
  point P4 (-82.3, -125.6)
  dimension "d159" = 5
  dimension "d160" = 5
  dimension "d161" = 5
  dimension "d162" = 5
  constraints: 2 horizontal alignment, 2 vertical alignment
  measures "d159" distance from line of L0 point (85.3, 64.858)
  measures "d160" distance from line of L2 point (85.3, 64.858)
  measures "d161" distance from line of L1 point (-82.3, 64.858)
  measures "d162" distance from line of L3 point (-82.3, -125.6)
hole "Agujero1" at (-82.3, 64.858, 0) at (85.3, 64.858, 0) at (85.3, -125.6, 0) at (-82.3, -125.6, 0) direction (0, 0, -1) diameter 3.3 end through all
sketch "Boceto4" plane through (0, 0, 0) normal (0, 0, 1) x (1, 0, 0)
  circle A0 centre (-82.3, 64.858) radius 1.65 construction
  circle A1 centre (85.3, 64.858) radius 1.65 construction
  circle A2 centre (85.3, -125.6) radius 1.65 construction
  circle A3 centre (-82.3, -125.6) radius 1.65 construction
  line L0 (-73.3, 65.858) -> (-71.3, 65.858)
  line L1 (-71.3, 65.858) -> (-71.3, 63.858)
  line L2 (-71.3, 63.858) -> (-73.3, 63.858)
  line L3 (-73.3, 63.858) -> (-73.3, 65.858)
  line L4 (-73.3, 65.858) -> (-71.3, 63.858) construction
  line L5 (-71.3, 65.858) -> (-73.3, 63.858) construction
  line L6 (-81.3, 55.858) -> (-83.3, 55.858)
  line L7 (-83.3, 55.858) -> (-83.3, 53.858)
  line L8 (-83.3, 53.858) -> (-81.3, 53.858)
  line L9 (-81.3, 53.858) -> (-81.3, 55.858)
  line L10 (-81.3, 55.858) -> (-83.3, 53.858) construction
  line L11 (-83.3, 55.858) -> (-81.3, 53.858) construction
  line L12 (76.3, 65.858) -> (74.3, 65.858)
  line L13 (74.3, 65.858) -> (74.3, 63.858)
  line L14 (74.3, 63.858) -> (76.3, 63.858)
  line L15 (76.3, 63.858) -> (76.3, 65.858)
  line L16 (76.3, 65.858) -> (74.3, 63.858) construction
  line L17 (74.3, 65.858) -> (76.3, 63.858) construction
  line L18 (86.3, 55.858) -> (84.3, 55.858)
  line L19 (84.3, 55.858) -> (84.3, 53.858)
  line L20 (84.3, 53.858) -> (86.3, 53.858)
  line L21 (86.3, 53.858) -> (86.3, 55.858)
  line L22 (86.3, 55.858) -> (84.3, 53.858) construction
  line L23 (84.3, 55.858) -> (86.3, 53.858) construction
  line L24 (84.3, -116.6) -> (86.3, -116.6)
  line L25 (86.3, -116.6) -> (86.3, -114.6)
  line L26 (86.3, -114.6) -> (84.3, -114.6)
  line L27 (84.3, -114.6) -> (84.3, -116.6)
  line L28 (84.3, -116.6) -> (86.3, -114.6) construction
  line L29 (86.3, -116.6) -> (84.3, -114.6) construction
  line L30 (74.3, -126.6) -> (76.3, -126.6)
  line L31 (76.3, -126.6) -> (76.3, -124.6)
  line L32 (76.3, -124.6) -> (74.3, -124.6)
  line L33 (74.3, -124.6) -> (74.3, -126.6)
  line L34 (74.3, -126.6) -> (76.3, -124.6) construction
  line L35 (76.3, -126.6) -> (74.3, -124.6) construction
  line L36 (-71.3, -126.6) -> (-73.3, -126.6)
  line L37 (-73.3, -126.6) -> (-73.3, -124.6)
  line L38 (-73.3, -124.6) -> (-71.3, -124.6)
  line L39 (-71.3, -124.6) -> (-71.3, -126.6)
  line L40 (-71.3, -126.6) -> (-73.3, -124.6) construction
  line L41 (-73.3, -126.6) -> (-71.3, -124.6) construction
  line L42 (-81.3, -114.6) -> (-83.3, -114.6)
  line L43 (-83.3, -114.6) -> (-83.3, -116.6)
  line L44 (-83.3, -116.6) -> (-81.3, -116.6)
  line L45 (-81.3, -116.6) -> (-81.3, -114.6)
  line L46 (-81.3, -114.6) -> (-83.3, -116.6) construction
  line L47 (-83.3, -114.6) -> (-81.3, -116.6) construction
  point P0 (0, 0)
  point P1 (-82.3, 54.858)
  point P2 (-72.3, 64.858)
  point P3 (75.3, 64.858)
  point P4 (85.3, 54.858)
  point P5 (85.3, -115.6)
  point P6 (75.3, -125.6)
  point P7 (-82.3, -115.6)
  point P8 (-72.3, -125.6)
  point P9 (-72.3, 64.858)
  point P10 (75.3, -125.6)
  dimension "d170" = 2
  dimension "d171" = 2
  dimension "d172" = 2
  dimension "d173" = 2
  dimension "d174" = 2
  dimension "d175" = 2
  dimension "d176" = 2
  dimension "d177" = 2
  dimension "d178" = 2
  dimension "d179" = 2
  dimension "d180" = 2
  dimension "d181" = 2
  dimension "d182" = 2
  dimension "d183" = 2
  dimension "d184" = 2
  dimension "d185" = 2
  dimension "d186" = 10
  dimension "d187" = 10
  dimension "d188" = 10
  dimension "d189" = 10
  dimension "d190" = 10
  dimension "d191" = 10
  dimension "d192" = 10
  dimension "d193" = 10
  constraints: 96 end point, 18 midpoint, 16 parallel, 8 horizontal, 8 perpendicular, 4 horizontal alignment, 4 vertical alignment
  measures "d170" distance of L1.end L2.end
  measures "d171" distance of L0.end L1.end
  measures "d172" distance of L8.end L7.end
  measures "d173" distance of L7.end L6.end
  measures "d174" distance of L14.end L13.end
  measures "d175" distance of L13.end L12.end
  measures "d176" distance of L20.end L19.end
  measures "d177" distance of L19.end L18.end
  measures "d178" distance of L26.end L25.end
  measures "d179" distance of L25.end L24.end
  measures "d180" distance of L32.end L31.end
  measures "d181" distance of L31.end L30.end
  measures "d182" distance of L37.end L38.end
  measures "d183" distance of L36.end L37.end
  measures "d184" distance of L44.end L43.end
  measures "d185" distance of L43.end L42.end
  measures "d186" distance of point (-82.3, -115.6) A3.centre
  measures "d187" distance of A3.centre point (-72.3, -125.6)
  measures "d188" distance of point (85.3, -115.6) A2.centre
  measures "d189" distance of A2.centre point (75.3, -125.6)
  measures "d190" distance of A1.centre point (75.3, 64.858)
  measures "d191" distance of A1.centre point (85.3, 54.858)
  measures "d192" distance of A0.centre point (-72.3, 64.858)
  measures "d193" distance of A0.centre point (-82.3, 54.858)
extrude "Extrusión3" add sketch "Boceto4" along normal blind 0.005
sketch "Boceto5" plane through (0, 0, 0.005) normal (0, 0, 1) x (1, 0, 0)
  line L0 (-71.3, 65.858) -> (-73.3, 65.858) construction
  line L1 (-73.3, 65.858) -> (-73.3, 63.858) construction
  line L2 (-73.3, 63.858) -> (-71.3, 63.858) construction
  line L3 (-71.3, 63.858) -> (-71.3, 65.858) construction
  line L4 (-81.3, 55.858) -> (-83.3, 55.858) construction
  line L5 (-83.3, 55.858) -> (-83.3, 53.858) construction
  line L6 (-83.3, 53.858) -> (-81.3, 53.858) construction
  line L7 (-81.3, 53.858) -> (-81.3, 55.858) construction
  line L8 (76.3, 65.858) -> (74.3, 65.858) construction
  line L9 (74.3, 65.858) -> (74.3, 63.858) construction
  line L10 (74.3, 63.858) -> (76.3, 63.858) construction
  line L11 (76.3, 63.858) -> (76.3, 65.858) construction
  line L12 (86.3, 55.858) -> (84.3, 55.858) construction
  line L13 (84.3, 55.858) -> (84.3, 53.858) construction
  line L14 (84.3, 53.858) -> (86.3, 53.858) construction
  line L15 (86.3, 53.858) -> (86.3, 55.858) construction
  line L16 (84.3, -116.6) -> (86.3, -116.6) construction
  line L17 (86.3, -116.6) -> (86.3, -114.6) construction
  line L18 (86.3, -114.6) -> (84.3, -114.6) construction
  line L19 (84.3, -114.6) -> (84.3, -116.6) construction
  line L20 (74.3, -126.6) -> (76.3, -126.6) construction
  line L21 (76.3, -126.6) -> (76.3, -124.6) construction
  line L22 (76.3, -124.6) -> (74.3, -124.6) construction
  line L23 (74.3, -124.6) -> (74.3, -126.6) construction
  line L24 (-73.3, -126.6) -> (-71.3, -126.6) construction
  line L25 (-71.3, -126.6) -> (-71.3, -124.6) construction
  line L26 (-71.3, -124.6) -> (-73.3, -124.6) construction
  line L27 (-73.3, -124.6) -> (-73.3, -126.6) construction
  line L28 (-81.3, -114.6) -> (-83.3, -114.6) construction
  line L29 (-83.3, -114.6) -> (-83.3, -116.6) construction
  line L30 (-83.3, -116.6) -> (-81.3, -116.6) construction
  line L31 (-81.3, -116.6) -> (-81.3, -114.6) construction
  circle A0 centre (-82.3, -115.6) radius 0.5
  circle A1 centre (-72.3, -125.6) radius 0.5
  circle A2 centre (75.3, -125.6) radius 0.5
  circle A3 centre (85.3, -115.6) radius 0.5
  circle A4 centre (85.3, 54.858) radius 0.5
  circle A5 centre (75.3, 64.858) radius 0.5
  circle A6 centre (-72.3, 64.858) radius 0.5
  circle A7 centre (-82.3, 54.858) radius 0.5
  circle A8 centre (-82.3, 64.858) radius 1.65 construction
  circle A9 centre (-82.3, -125.6) radius 1.65 construction
  circle A10 centre (85.3, -125.6) radius 1.65 construction
  circle A11 centre (85.3, 64.858) radius 1.65 construction
  point P0 (0, 0)
  dimension "d196" = 1
  dimension "d197" = 1
  dimension "d198" = 1
  dimension "d199" = 1
  dimension "d200" = 1
  dimension "d201" = 1
  dimension "d202" = 1
  dimension "d203" = 1
  dimension "d204" = 10
  dimension "d205" = 10
  dimension "d206" = 10
  dimension "d207" = 10
  dimension "d208" = 10
  dimension "d209" = 10
  dimension "d210" = 10
  dimension "d211" = 10
  constraints: 8 centre point, 4 horizontal alignment, 4 vertical alignment
  measures "d196" diameter of A0
  measures "d197" diameter of A1
  measures "d198" diameter of A2
  measures "d199" diameter of A3
  measures "d200" diameter of A4
  measures "d201" diameter of A5
  measures "d202" diameter of A6
  measures "d203" diameter of A7
  measures "d204" distance of A6.centre A8.centre
  measures "d205" distance of A8.centre A7.centre
  measures "d206" distance of A5.centre A11.centre
  measures "d207" distance of A11.centre A4.centre
  measures "d208" distance of A3.centre A10.centre
  measures "d209" distance of A10.centre A2.centre
  measures "d210" distance of A9.centre A1.centre
  measures "d211" distance of A9.centre A0.centre
extrude "Extrusión4" add sketch "Boceto5" along normal blind 0.005
ref_plane "Plano de trabajo1" through (0, 0, -0.871) normal (0, 0, 1) x (1, 0, 0)
mirror "Simetría2" about plane through (0, 0, -0.871) normal (0, 0, 1) of "Extrusión3"
mirror "Simetría3" about plane through (0, 0, -0.871) normal (0, 0, 1) of "Extrusión4"
sketch "Boceto6" plane through (0, 0, 0) normal (0, 0, 1) x (1, 0, 0)
  line L0 (90.3, -130.6) -> (-87.3, -130.6) construction
  point P0 (0, 0)
  point P1 (-55.3, 51.4)
  point P2 (-55.3, -8.6)
  point P3 (-55.3, -98.6)
  point P4 (58.3, -98.6)
  point P5 (58.3, -43.6)
  point P6 (58.3, 11.4)
  dimension "d214" = 55
  dimension "d215" = 55
  dimension "d216" = 32
  dimension "d217" = 32
  dimension "d218" = 90
  dimension "d219" = 60
  dimension "d220" = 32
  dimension "d221" = 32
  constraints: 4 vertical alignment
  measures "d214" distance of point (58.3, -43.6) point (58.3, -98.6)
  measures "d215" distance of point (58.3, 11.4) point (58.3, -43.6)
  measures "d216" distance from line of L0 point (58.3, -98.6)
  measures "d217" distance from line of L0 point (-55.3, -98.6)
  measures "d218" distance of point (-55.3, -8.6) point (-55.3, -98.6)
  measures "d219" distance of point (-55.3, 51.4) point (-55.3, -8.6)
  measures "d220" horizontal distance of L0.start point (58.3, -98.6)
  measures "d221" horizontal distance of L0.end point (-55.3, -98.6)
hole "Agujero2" at (-55.3, 51.4, 0) at (-55.3, -8.6, 0) at (-55.3, -98.6, 0) at (58.3, -98.6, 0) at (58.3, -43.6, 0) at (58.3, 11.4, 0) direction (0, 0, -1) diameter 3.3 depth 1.742 tip angle 118 countersink diameter 5.6 countersink angle 90
fillet "Empalme1" radius 0.5 1 edges at (-28, 27.342, -0.871)
